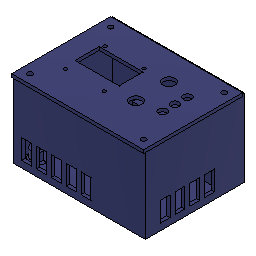
SensorUnit housing v20 (Autodesk Fusion 360 design; units mm, degrees)
Autodesk Fusion 360 part; units mm, degrees
sketch "Sketch1" plane through (0, 0, 0) normal (0, 1, 0) x (1, 0, 0)
  line L0 (26, -8.5) -> (-26, -8.5)
  line L1 (-26, -8.5) -> (-26, 8.5)
  line L2 (-26, 8.5) -> (26, 8.5)
  line L3 (26, 8.5) -> (26, -8.5)
  line L4 (26, -8.5) -> (-26, 8.5) construction
  line L5 (-26, -8.5) -> (26, 8.5) construction
  line L6 (15, -1) -> (-15, -1)
  line L7 (-15, -1) -> (-15, 1)
  line L8 (-15, 1) -> (15, 1)
  line L9 (15, 1) -> (15, -1)
  line L10 (15, -1) -> (-15, 1) construction
  line L11 (-15, -1) -> (15, 1) construction
  circle A0 centre (15, 0) radius 3.365
  circle A1 centre (-15, 0) radius 3.365
  dimension "d1" = 52
  dimension "d2" = 17
  dimension "d3" = 6.73
  dimension "d4" = 6.73
  constraint horizontal L0
  constraint perpendicular L0 L1
  constraint parallel L0 L2
  constraint parallel L1 L3
  constraint coincident L4 origin
  constraint coincident L5 origin
  constraint horizontal L6
  constraint perpendicular L6 L7
  constraint parallel L6 L8
  constraint parallel L7 L9
  constraint coincident L10 origin
  constraint coincident L11 origin
  constraint midpoint L9 A0.centre
  constraint midpoint L7 A1.centre
  measures "d1" distance of L1.end L2.end
  measures "d2" distance of L0.start L2.end
  measures "d3" diameter of A0
  measures "d4" diameter of A1
sketch "Sketch2" plane through (0, 0, 0) normal (0, 1, 0) x (1, 0, 0)
  line L0 (40, -30) -> (-40, -30)
  line L1 (-40, -30) -> (-40, 30)
  line L2 (-40, 30) -> (40, 30)
  line L3 (40, 30) -> (40, -30)
  line L4 (40, -30) -> (-40, 30) construction
  line L5 (-40, -30) -> (40, 30) construction
  line L6 (26, -14) -> (-26, -14) construction
  line L7 (-26, -14) -> (-26, 14) construction
  line L8 (-26, 14) -> (26, 14) construction
  line L9 (26, 14) -> (26, -14) construction
  line L10 (26, -14) -> (-26, 14) construction
  line L11 (-26, -14) -> (26, 14) construction
  line L12 (1.4523, -7.9433) -> (-23.5477, -7.9433) construction
  line L13 (-23.5477, -7.9433) -> (-23.5477, 8.0567) construction
  line L14 (-23.5477, 8.0567) -> (1.4523, 8.0567) construction
  line L15 (1.4523, 8.0567) -> (1.4523, -7.9433) construction
  line L16 (1.4523, -7.9433) -> (-23.5477, 8.0567) construction
  line L17 (-23.5477, -7.9433) -> (1.4523, 8.0567) construction
  point P0 (-11.0477, 0.0567)
  dimension "d7" = 80
  dimension "d8" = 60
  dimension "d9" = 52
  dimension "d10" = 28
  dimension "d11" = 25
  dimension "d12" = 16
  constraint horizontal L0
  constraint perpendicular L0 L1
  constraint parallel L0 L2
  constraint parallel L1 L3
  constraint coincident L4 origin
  constraint coincident L5 origin
  constraint horizontal L6
  constraint perpendicular L6 L7
  constraint parallel L6 L8
  constraint parallel L7 L9
  constraint coincident L10 origin
  constraint coincident L11 origin
  constraint horizontal L12
  constraint perpendicular L12 L13
  constraint parallel L12 L14
  constraint parallel L13 L15
  constraint coincident L16 P0
  constraint coincident L17 P0
  measures "d7" distance of L1.end L2.end
  measures "d8" distance of L0.start L2.end
  measures "d9" distance of L7.end L8.end
  measures "d10" distance of L6.end L7.end
  measures "d11" distance of L13.end L14.end
  measures "d12" distance of L12.end L13.end
extrude "Extrude2" add sketch "Sketch2" along normal blind 2.5 makes body 1
sketch "Sketch3" plane through (0, 2.5, 0) normal (0, 1, 0) x (-1, 0, 0)
  line L0 (-40, -30) -> (40, -30)
  line L1 (40, -30) -> (40, 30)
  line L2 (40, 30) -> (-40, 30)
  line L3 (-40, 30) -> (-40, -30)
  line L4 (40, -30) -> (-40, 30) construction
  line L5 (-40, -30) -> (40, 30) construction
  line L6 (-16.7, 25) -> (35, 25)
  line L7 (35, 25) -> (35, -3)
  line L8 (35, -3) -> (-16.7, -3)
  line L9 (-16.7, -3) -> (-16.7, 25)
  line L10 (-16.7, 25) -> (35, -3) construction
  line L11 (35, 25) -> (-16.7, -3) construction
  circle A0 centre (32.7, -0.7) radius 2.3971
  line L12 (9.15, -3) -> (9.15, 25) construction
  line L13 (35, 11) -> (-16.7, 11) construction
  circle A1 centre (32.7, 22.7) radius 2.3971
  circle A2 centre (-14.4, -0.7) radius 2.3971
  circle A3 centre (-14.4, 22.7) radius 2.3971
  circle A4 centre (32.7, -0.7) radius 3.8971
  circle A5 centre (32.7, 22.7) radius 3.8971
  circle A6 centre (-14.4, -0.7) radius 3.8971
  circle A7 centre (-14.4, 22.7) radius 3.8971
  point P0 (9.15, 11)
  dimension "d18" = 51.7
  dimension "d22" = 28
  dimension "d23" = 2.3
  dimension "d24" = 2.3
  dimension "d25" = 5
  dimension "d26" = 5
  dimension "d27" = 1.5
  constraint coincident L0.end L1.start
  constraint coincident L2.end L3.start
  constraint coincident L0.start L3.end
  constraint coincident L1.end L2.start
  constraint horizontal L6
  constraint perpendicular L6 L7
  constraint parallel L6 L8
  constraint parallel L7 L9
  constraint coincident L10 P0
  constraint coincident L11 P0
  constraint midpoint L8 L12.start
  constraint midpoint L6 L12.end
  constraint midpoint L7 L13.start
  constraint midpoint L9 L13.end
  constraint symmetric A0 L13 A1
  constraint symmetric A0 L12 A2
  constraint symmetric L12 A1 A3
  constraint concentric A0 A4
  constraint symmetric L13 A4 A5
  constraint symmetric L12 A4 A6
  constraint symmetric L12 A5 A7
  measures "d18" distance of L7.end L8.end
  measures "d22" distance of L6.start L8.end
  measures "d23" distance of L8 A0.centre
  measures "d24" distance of L7 A0.centre
  measures "d25" distance of L1 L7
  measures "d26" distance of L2 L6
  measures "d27" distance of A0 A4
extrude "Extrude4" cut sketch "Sketch3" against normal up to surface (2 mm away) from surface at -0.5 contours L6 L9 A3 A7 | L6 L9 A3 | L6 A3 | L6 L9 A3 | L9 A3 | L6 L9 A3 A7 | L6 L7 A1 A5 | L6 L7 A1 A5 | L8 L9 A2 A6 | L8 L9 A2 A6 | L6 A1 | L6 L7 A1 | L8 L9 A2 | L9 A2 | L6 L7 A1 | L7 A1 | L7 L8 A0 A4 | L7 L8 A0 A4 | L8 L9 A2 | L8 A2 | L7 A0 | L7 L8 A0 | L8 A0 | L7 L8 A0 bodies 1
extrude "Extrude5" cut sketch "Sketch3" against normal up to surface (0.5 mm away) contours L6 A3 | L6 L9 A3 | L9 A3 | L6 A1 | L6 L7 A1 | L8 L9 A2 | L9 A2 | L7 A1 | L8 A2 | L7 A0 | L7 L8 A0 | L8 A0 picked at (-15.1667, 23.1388) picked at (32.4467, 23.7731) picked at (-13.7719, -0.5156) picked at (33.3362, -0.4496) bodies 1
extrude "Extrude6" add sketch "Sketch3" along normal blind 6.5 from surface at -0.5 contours L6 L9 A3 A7 | L6 L9 A3 | L6 L9 A3 A7 | L6 L7 A1 A5 | L6 L7 A1 A5 | L8 L9 A2 A6 | L8 L9 A2 A6 | L6 L7 A1 | L7 L8 A0 A4 | L7 L8 A0 A4 | L8 L9 A2 | L7 L8 A0 picked at (-16.2938, 24.5938) picked at (34.5938, 24.5938) picked at (-16.2938, -2.5938) picked at (34.5938, -2.5938) bodies 1
chamfer "Chamfer1" distance 1 angle 45 1 edges at (-29.0666, 2.5, 0.7092) on bodies 1
chamfer "Chamfer1" distance 1 angle 45 3 edges at (-29.0666, 2.5, 24.1092) (18.0334, 2.5, 24.1092) (18.0334, 2.5, 0.7092) on bodies 1
sketch "Sketch4" plane through (0, 2.5, 0) normal (0, 1, 0) x (-1, 0, 0)
  line L0 (-38, 28) -> (38, 28)
  line L1 (38, 28) -> (38, -28)
  line L2 (38, -28) -> (-38, -28)
  line L3 (-38, -28) -> (-38, 28)
  line L4 (-38, 28) -> (38, -28) construction
  line L5 (38, 28) -> (-38, -28) construction
  line L6 (-40, -30) -> (40, -30)
  line L7 (40, 30) -> (-40, 30)
  line L8 (-40, 30) -> (-40, -30)
  line L9 (40, -30) -> (40, 30)
  line L10 (30, 8.5) -> (38, 8.5) construction
  dimension "d42" = 2
  dimension "d43" = 2
  dimension "d44" = 2
  dimension "d45" = 2
  constraint horizontal L0
  constraint perpendicular L0 L1
  constraint parallel L0 L2
  constraint parallel L1 L3
  constraint coincident L4 origin
  constraint coincident L5 origin
  constraint coincident L1 L10.end
  constraint perpendicular L1 L10
  measures "d42" distance of L1 L9
  measures "d43" distance of L3 L8
  measures "d44" distance of L2 L6
  measures "d45" distance of L0 L7
sketch "Sketch18" plane through (0, 2.5, 0) normal (0, 1, 0) x (-1, 0, 0)
  circle A0 centre (-14.4, 22.7) radius 4.8971
  circle A1 centre (32.7, -0.7) radius 4.8971
  line L0 (-40, -30) -> (40, -30)
  line L1 (40, -30) -> (40, 30)
  line L2 (40, 30) -> (-40, 30)
  line L3 (-40, 30) -> (-40, -30)
  circle A2 centre (32.7, 22.7) radius 4.8971
  circle A3 centre (-14.4, -0.7) radius 4.8971
  line L4 (32.7, -0.7) -> (32.7, 0.8) construction
  line L5 (32.7, 0.8) -> (28.0383, 0.8)
  line L6 (32.7, 0.8) -> (28.0383, 0.8)
  line L7 (32.7, 22.7) -> (32.7, 21.2) construction
  line L8 (32.7, 21.2) -> (28.0383, 21.2)
  line L9 (32.7, 21.2) -> (28.0383, 21.2)
  line L10 (32.7, 22.7) -> (27.8029, 22.7)
  line L11 (32.7, 22.7) -> (37.5971, 22.7)
  line L12 (32.7, -0.7) -> (27.8029, -0.7)
  line L13 (32.7, -0.7) -> (37.5971, -0.7)
  dimension "d140" = 1.5
  dimension "d141" = 1.5
  constraint coincident A1.centre L4.start
  constraint vertical L4
  constraint coincident A1 L5.end
  constraint perpendicular L4 L5
  constraint perpendicular L4 L6
  constraint coincident A2.centre L7.start
  constraint perpendicular L6 L7
  constraint coincident A2 L8.end
  constraint perpendicular L7 L8
  constraint perpendicular L7 L9
  constraint coincident A2 L10.end
  constraint perpendicular L7 L10
  constraint coincident A2 L11.end
  constraint perpendicular L7 L11
  constraint coincident A1 L12.end
  constraint perpendicular L4 L12
  constraint coincident A1 L13.end
  constraint perpendicular L4 L13
  measures "d140" distance of A1.centre L4.end
  measures "d141" distance of A2.centre L7.end
extrude "Extrude21" cut sketch "Sketch18" along normal up to surface (6 mm away) contours A1 L12 L13 | A2 L10 L11 picked at (32.7218, 2.5556) picked at (32.7218, 19.4444) bodies 1
extrude "Extrude7" add sketch "Sketch4" along normal blind 45 from surface at -0.5 bodies 1
sketch "Sketch5" plane through (0, 2.5, 0) normal (0, 1, 0) x (-1, 0, 0)
  line L0 (-38, -28) -> (13, -28)
  line L1 (13, -28) -> (13, -17)
  line L2 (13, -17) -> (-38, -17)
  line L3 (-38, -17) -> (-38, -28)
  line L4 (-38, -28) -> (14, -28)
  line L5 (14, -28) -> (14, -16)
  line L6 (14, -16) -> (-38, -16)
  line L7 (-38, -16) -> (-38, -28)
  line L8 (-40, 30) -> (-40, -30)
  line L9 (-40, -30) -> (40, -30)
  dimension "d49" = 51
  dimension "d50" = 11
  dimension "d51" = 1
  dimension "d52" = 1
  dimension "d215" = 2
  dimension "d216" = 2
  constraint horizontal L0
  constraint vertical L1
  constraint horizontal L2
  constraint vertical L3
  constraint horizontal L4
  constraint vertical L5
  constraint horizontal L6
  constraint vertical L7
  measures "d49" distance of L1.end L2.end
  measures "d50" distance of L0.end L1.end
  measures "d51" distance of L2 L6
  measures "d52" distance of L1 L5
  measures "d215" distance of L3 L8
  measures "d216" distance of L4 L9
extrude "Extrude8" add sketch "Sketch5" along normal blind 20 from surface at -0.5 contours L1 L2 L4 L5 L6 L7 bodies 1
sketch "Sketch6" plane through (0, 0, -28) normal (0, 0, 1) x (1, 0, 0)
  line L0 (-13, 2.5) -> (38, 2.5)
  line L1 (38, 2.5) -> (38, 47)
  line L2 (38, 47) -> (-38, 47)
  line L3 (-38, 47) -> (-38, 2.5)
  line L4 (38, 2.5) -> (-13, 2.5)
  line L5 (-13, 2.5) -> (-13, 22)
  line L6 (-13, 22) -> (38, 22)
  line L7 (38, 22) -> (38, 2.5)
  line L8 (36.5, 4) -> (-11.5, 4)
  line L9 (-11.5, 4) -> (-11.5, 20)
  line L10 (-11.5, 20) -> (36.5, 20)
  line L11 (36.5, 20) -> (36.5, 4)
  line L12 (-13, 22) -> (-13, 2.5)
  line L13 (-38, 2.5) -> (-14, 2.5)
  line L14 (-14, 2.5) -> (-14, 22)
  line L15 (-14, 22) -> (-13, 22)
  dimension "d56" = 1.5
  dimension "d57" = 1.5
  dimension "d58" = 1.5
  dimension "d59" = 16
  constraint horizontal L4
  constraint vertical L5
  constraint horizontal L6
  constraint vertical L7
  constraint coincident L0.end L1.start
  constraint horizontal L8
  constraint vertical L9
  constraint horizontal L10
  constraint vertical L11
  measures "d56" distance of L4 L8
  measures "d57" distance of L7 L11
  measures "d58" distance of L5 L9
  measures "d59" distance of L8 L10
extrude "Extrude9" cut sketch "Sketch6" against normal up to surface (2 mm away) contours L8 L9 L10 L11 bodies 1
sketch "Sketch7" plane through (0, 22, 0) normal (0, 1, 0) x (-1, 0, 0)
  line L0 (14, -28) -> (14, -16)
  line L1 (14, -16) -> (-38, -16)
  line L2 (-38, -17) -> (13, -17)
  line L3 (13, -17) -> (13, -28)
  line L4 (13, -25.5) -> (14, -25.5)
  line L5 (14, -25.5) -> (14, -17)
  line L6 (14, -17) -> (13, -17)
  line L7 (13, -17) -> (13, -25.5)
  line L8 (14, -16) -> (-38, -16)
  line L9 (-38, -16) -> (-38, -28)
  line L10 (-38, -28) -> (14, -28)
  line L11 (14, -28) -> (14, -16)
  line L12 (13, -28) -> (14, -28)
  line L13 (-38, -16) -> (-38, -17)
  line L14 (-40, -30) -> (40, -30)
  line L15 (-40, 30) -> (-40, -30)
  dimension "d63" = 8.5
  dimension "d217" = 2
  dimension "d218" = 2
  constraint horizontal L4
  constraint vertical L5
  constraint horizontal L6
  constraint vertical L7
  constraint coincident L0 L5.end
  constraint coincident L3 L4.start
  constraint horizontal L8
  constraint vertical L9
  constraint horizontal L10
  constraint vertical L11
  constraint coincident L0.end L1.start
  measures "d63" distance of L4.start L2.end
  measures "d217" distance of L10 L14
  measures "d218" distance of L9 L15
extrude "Extrude11" add sketch "Sketch7" along normal blind 1 from surface at -0.5 bodies 1
extrude "Extrude10" cut sketch "Sketch7" against normal blind 4 from surface at -0.5 contours L0 L3 L4 L5 L6 L7 L11 bodies 1
sketch "Sketch9" plane through (-38, 0, 0) normal (1, 0, 0) x (0, 0, -1)
  line L0 (-28, 2.5) -> (28, 2.5)
  line L1 (28, 2.5) -> (28, 47)
  line L2 (28, 47) -> (-28, 47)
  line L3 (-28, 47) -> (-28, 2.5)
  line L4 (-4.5, 3.5) -> (-17.5, 3.5)
  line L5 (-17.5, 3.5) -> (-17.5, 13.5)
  line L6 (-17.5, 13.5) -> (-4.5, 13.5)
  line L7 (-4.5, 13.5) -> (-4.5, 3.5)
  line L8 (-4.5, 3.5) -> (-17.5, 13.5) construction
  line L9 (-17.5, 3.5) -> (-4.5, 13.5) construction
  line L10 (-30, 0) -> (-30, 47)
  line L11 (-28, 2.5) -> (28, 2.5)
  point P0 (-11, 8.5)
  dimension "d71" = 19
  dimension "d72" = 6
  dimension "d73" = 10
  dimension "d74" = 13
  constraint horizontal L4
  constraint perpendicular L4 L5
  constraint parallel L4 L6
  constraint parallel L5 L7
  constraint coincident L8 P0
  constraint coincident L9 P0
  measures "d71" distance of P0 L10
  measures "d72" distance of P0 L11
  measures "d73" distance of L4 L6
  measures "d74" distance of L5.end L6.end
extrude "Extrude12" cut sketch "Sketch9" against normal up to surface (2 mm away) contours L4 L5 L6 L7 bodies 1
sketch "Sketch10" plane through (0, 47, 0) normal (0, 1, 0) x (-1, 0, 0)
  line L0 (38, -28) -> (-38, -28)
  line L1 (-38, -28) -> (-38, 28)
  line L2 (-38, 28) -> (38, 28)
  line L3 (38, 28) -> (38, -28)
  line L4 (40, -30) -> (40, 30)
  line L5 (40, 30) -> (-40, 30)
  line L6 (-40, 30) -> (-40, -30)
  line L7 (-40, -30) -> (40, -30)
  line L8 (-38, -28) -> (-30.9289, -20.9289)
  line L9 (-38, -28) -> (-23, -28) construction
  line L10 (-30.9289, -20.9289) -> (-38, -13.8579)
  line L11 (-30.9289, -20.9289) -> (-35.9289, -20.9289) construction
  line L12 (-30.9289, -20.9289) -> (-23.8579, -28)
  line L13 (0, -28) -> (0, 28) construction
  line L14 (-38, 28) -> (38, -28) construction
  line L15 (38, 0) -> (-38, 0) construction
  line L16 (-30.9289, 20.9289) -> (-38, 13.8579)
  line L17 (-30.9289, 20.9289) -> (-23.8579, 28)
  line L18 (30.9289, -20.9289) -> (38, -13.8579)
  line L19 (30.9289, -20.9289) -> (23.8579, -28)
  line L20 (30.9289, 20.9289) -> (38, 13.8579)
  line L21 (30.9289, 20.9289) -> (23.8579, 28)
  circle A0 centre (-34.4645, -24.4645) radius 1.5
  circle A1 centre (-34.4645, 24.4645) radius 1.5
  circle A2 centre (34.4645, -24.4645) radius 1.5
  circle A3 centre (34.4645, 24.4645) radius 1.5
  dimension "d78" = 45
  dimension "d79" = 10
  dimension "d80" = 45
  dimension "d81" = 180
  dimension "d85" = 3
  dimension "d86" = 5
  constraint horizontal L9
  constraint coincident L0.end L1.start
  constraint horizontal L11
  constraint coincident L1 L10.end
  constraint coincident L0 L12.end
  constraint midpoint L0 L13.start
  constraint midpoint L2 L13.end
  constraint coincident L1.end L2.start
  constraint coincident L0.start L3.end
  constraint midpoint L3 L15.start
  constraint midpoint L1 L15.end
  constraint symmetric L8.end L15 L16.start
  constraint symmetric L10.end L15 L16.end
  constraint symmetric L12.end L15 L17.end
  constraint symmetric L8.end L13 L18.start
  constraint symmetric L10.end L13 L18.end
  constraint symmetric L12.end L13 L19.end
  constraint symmetric L13 L16.start L20.start
  constraint symmetric L13 L16.end L20.end
  constraint symmetric L13 L17.end L21.end
  constraint coincident L8 A0.centre
  constraint symmetric L15 A0 A1
  constraint symmetric L13 A0 A2
  constraint symmetric L13 A1 A3
  measures "d78" angle of L8 L9
  measures "d79" distance of L0.end L8.end
  measures "d80" angle of L10 L11
  measures "d81" angle of L10 L12
  measures "d85" diameter of A0
  measures "d86" distance of L0.end A0.centre
extrude "Extrude13" add sketch "Sketch10" against normal blind 3 contours L0 L3 L18 L19 | L0 L8 L12 A0 | L2 L3 L20 L21 | L1 L8 L10 A0 | L8 A0 | L8 A0 | L1 L2 L16 L17 | A1 | A2 | A3 bodies 1
extrude "Extrude14" cut sketch "Sketch10" against normal up to surface (3 mm away) contours L8 A0 | L8 A0 | A1 | A2 | A3 bodies 1
sketch "Sketch11" plane through (0, 47, 0) normal (0, 1, 0) x (-1, 0, 0)
  line L0 (38.6239, -27.551) -> (-41.3761, -27.551)
  line L1 (-41.3761, -27.551) -> (-41.3761, 32.449)
  line L2 (-41.3761, 32.449) -> (38.6239, 32.449)
  line L3 (38.6239, 32.449) -> (38.6239, -27.551)
  line L4 (-1.3761, -27.551) -> (-1.3761, 32.449) construction
  line L5 (-41.3761, 2.449) -> (38.6239, 2.449) construction
  line L6 (36.6239, -25.551) -> (40.6239, -25.551) construction
  line L7 (40.6239, -25.551) -> (40.6239, -29.551) construction
  line L8 (40.6239, -29.551) -> (36.6239, -29.551) construction
  line L9 (36.6239, -29.551) -> (36.6239, -25.551) construction
  line L10 (36.6239, -25.551) -> (40.6239, -29.551) construction
  line L11 (40.6239, -25.551) -> (36.6239, -29.551) construction
  line L12 (36.6239, -25.551) -> (33.0884, -22.0155) construction
  line L13 (36.6239, -25.551) -> (28, -25.551) construction
  circle A0 centre (33.0884, -22.0155) radius 1.5
  circle A1 centre (-35.8405, -22.0155) radius 1.5
  circle A2 centre (-35.8405, 26.9134) radius 1.5
  circle A3 centre (33.0884, 26.9134) radius 1.5
  point P0 (38.6239, -27.551)
  dimension "d91" = 80
  dimension "d92" = 60
  dimension "d93" = 2
  dimension "d94" = 2
  dimension "d95" = 45
  dimension "d96" = 5
  dimension "d97" = 3
  constraint horizontal L0
  constraint vertical L1
  constraint horizontal L2
  constraint vertical L3
  constraint midpoint L0 L4.start
  constraint midpoint L2 L4.end
  constraint midpoint L1 L5.start
  constraint midpoint L3 L5.end
  constraint horizontal L6
  constraint perpendicular L6 L7
  constraint parallel L6 L8
  constraint parallel L7 L9
  constraint coincident L10 P0
  constraint coincident L11 P0
  constraint coincident P0 L0.start
  constraint horizontal L13
  constraint coincident L12.end A0.centre
  constraint symmetric L4 A0 A1
  constraint symmetric L5 A0 A3
  constraint symmetric L5 A1 A2
  measures "d91" distance of P0 L0.end
  measures "d92" distance of P0 L2.end
  measures "d93" distance of L3 L9
  measures "d94" distance of L0 L6
  measures "d95" angle of L12 L13
  measures "d96" distance of L6.start L12.end
  measures "d97" diameter of A0
extrude "Extrude15" add sketch "Sketch11" along normal blind 2 separate body makes body 2
sketch "Sketch12" plane through (0, 49, 0) normal (0, 1, 0) x (-1, 0, 0)
  circle A0 centre (33.0884, 26.9134) radius 1.5
  circle A1 centre (-35.8405, 26.9134) radius 1.5
  circle A2 centre (33.0884, -22.0155) radius 1.5
  circle A3 centre (-35.8405, -22.0155) radius 1.5
  line L0 (38.6239, 32.449) -> (-41.3761, 32.449)
  line L1 (-41.3761, 32.449) -> (-41.3761, -27.551)
  line L2 (-41.3761, -27.551) -> (38.6239, -27.551)
  line L3 (38.6239, -27.551) -> (38.6239, 32.449)
  line L4 (-0.35, 6.3) -> (26.35, 6.3)
  line L5 (26.35, 6.3) -> (26.35, -8.3)
  line L6 (26.35, -8.3) -> (-0.35, -8.3)
  line L7 (-0.35, -8.3) -> (-0.35, 6.3)
  line L8 (-0.35, 6.3) -> (26.35, -8.3) construction
  line L9 (26.35, 6.3) -> (-0.35, -8.3) construction
  line L10 (-0.7, 15.6) -> (26.7, 15.6) construction
  line L11 (26.7, 15.6) -> (26.7, -12.3) construction
  line L12 (26.7, -12.3) -> (-0.7, -12.3) construction
  line L13 (-0.7, -12.3) -> (-0.7, 15.6) construction
  line L14 (-0.7, 15.6) -> (26.7, -12.3) construction
  line L15 (26.7, 15.6) -> (-0.7, -12.3) construction
  line L16 (13, -12.3) -> (13, 15.6) construction
  circle A4 centre (1.3, -10.3) radius 1
  circle A5 centre (24.7, -10.3) radius 1
  line L17 (-0.7, 1.65) -> (26.7, 1.65) construction
  circle A6 centre (24.7, 13.6) radius 1
  circle A7 centre (1.3, 13.6) radius 1
  point P0 (13, -1)
  point P1 (13, 1.65)
  dimension "d101" = 14.6
  dimension "d102" = 26.7
  dimension "d103" = 27.4
  dimension "d104" = 27.9
  dimension "d105" = 4
  dimension "d106" = 2
  dimension "d107" = 2
  dimension "d108" = 2
  constraint horizontal L4
  constraint perpendicular L4 L5
  constraint parallel L4 L6
  constraint parallel L5 L7
  constraint coincident L8 P0
  constraint coincident L9 P0
  constraint horizontal L10
  constraint perpendicular L10 L11
  constraint parallel L10 L12
  constraint parallel L11 L13
  constraint coincident L14 P1
  constraint coincident L15 P1
  constraint midpoint L12 L16.start
  constraint midpoint L10 L16.end
  constraint coincident P0 L16
  constraint symmetric L16 A4 A5
  constraint midpoint L13 L17.start
  constraint midpoint L11 L17.end
  constraint symmetric A4 L17 A7
  constraint symmetric A5 L17 A6
  measures "d101" distance of L4.start L6.end
  measures "d102" distance of L4.start L4.end
  measures "d103" distance of L11.end L12.end
  measures "d104" distance of L10.start L12.end
  measures "d105" distance of L6 L12
  measures "d106" diameter of A4
  measures "d107" distance of L12 A4.centre
  measures "d108" distance of L13 A4.centre
extrude "Extrude16" cut sketch "Sketch12" against normal up to surface (2 mm away) contours L4 L5 L6 L7 | A4 | A5 | A6 | A7 bodies 2
sketch "Sketch13" plane through (0, 2.5, 0) normal (0, 1, 0) x (-1, 0, 0)
  circle A0 centre (-13.35, -11) radius 3.65
  circle A1 centre (-13.35, 9) radius 3.65
  line L0 (-0.35, -8.3) -> (-0.35, 6.3)
  line L1 (-0.35, -1) -> (-38.1982, -1) construction
  dimension "d112" = 7.3
  dimension "d113" = 7.3
  dimension "d114" = 20
  dimension "d115" = 13
  dimension "d116" = 10
  constraint midpoint L0 L1.start
  constraint perpendicular L0 L1
  measures "d112" diameter of A1
  measures "d113" diameter of A0
  measures "d114" distance of A0.centre A1.centre
  measures "d115" distance of A0.centre L0
  measures "d116" distance of A0.centre L1
extrude "Extrude17" cut sketch "Sketch13" along normal up to surface (46.5 mm away) bodies 2
sketch "Sketch14" plane through (0, 0, -17) normal (0, 0, -1) x (-1, 0, 0)
  line L0 (13, 21.5) -> (-38, 21.5)
  line L1 (-38, 2.5) -> (13, 2.5)
  line L2 (13, 2.5) -> (13, 17)
  circle A0 centre (-33.5, 11.5) radius 1
  line L3 (11.5, 4) -> (-36.5, 4)
  line L4 (-36.5, 4) -> (-36.5, 20)
  line L5 (-38, 21.5) -> (-38, 2.5)
  line L6 (13, 17) -> (14, 17)
  line L7 (14, 17) -> (14, 21)
  line L8 (14, 21) -> (13, 21)
  line L9 (13, 21) -> (13, 21.5)
  dimension "d120" = 2
  dimension "d121" = 7.5
  dimension "d122" = 3
  measures "d120" diameter of A0
  measures "d121" distance of A0.centre L3
  measures "d122" distance of A0.centre L4
extrude "Extrude18" cut sketch "Sketch14" against normal up to surface (1 mm away) contours A0 bodies 1
sketch "Sketch16" plane through (0, 49, 0) normal (0, 1, 0) x (-1, 0, 0)
  circle A0 centre (-13.35, 9) radius 3.65
  circle A1 centre (-13.35, -11) radius 3.65
  circle A2 centre (24.7, -10.3) radius 1
  circle A3 centre (1.3, -10.3) radius 1
  circle A4 centre (24.7, 13.6) radius 1
  line L0 (-0.35, -8.3) -> (-0.35, 6.3)
  line L1 (-0.35, 6.3) -> (26.35, 6.3)
  line L2 (26.35, 6.3) -> (26.35, -8.3)
  line L3 (26.35, -8.3) -> (-0.35, -8.3)
  circle A5 centre (1.3, 13.6) radius 1
  circle A6 centre (33.0884, 26.9134) radius 1.5
  circle A7 centre (-35.8405, 26.9134) radius 1.5
  circle A8 centre (33.0884, -22.0155) radius 1.5
  circle A9 centre (-35.8405, -22.0155) radius 1.5
  line L4 (38.6239, 32.449) -> (-41.3761, 32.449)
  line L5 (-41.3761, 32.449) -> (-41.3761, -27.551)
  line L6 (-41.3761, -27.551) -> (38.6239, -27.551)
  line L7 (38.6239, -27.551) -> (38.6239, 32.449)
  line L8 (-27, -13.193) -> (-27, 11.193) construction
  circle A10 centre (-27, -1) radius 2.5
  circle A11 centre (-27, -8.5) radius 2.5
  circle A12 centre (-27, 6.5) radius 2.5
  dimension "d133" = 5
  dimension "d134" = 5
  dimension "d135" = 5
  dimension "d136" = 7.5
  dimension "d137" = 7.5
  constraint vertical L8
  constraint midpoint L8 A10.centre
  constraint coincident L8 A11.centre
  constraint coincident L8 A12.centre
  measures "d133" diameter of A10
  measures "d134" diameter of A11
  measures "d135" diameter of A12
  measures "d136" distance of A10.centre A12.centre
  measures "d137" distance of A10.centre A11.centre
extrude "Extrude20" cut sketch "Sketch16" against normal up to surface (2 mm away) contours A10 | A11 | A12 bodies 2
sketch "Sketch19" plane through (40, 0, 0) normal (1, 0, 0) x (0, 0, -1)
  line L0 (-30, 47) -> (-30, 0)
  line L1 (-30, 0) -> (30, 0)
  line L2 (30, 0) -> (30, 47)
  line L3 (30, 47) -> (-30, 47)
  line L4 (30, 10) -> (-30, 10) construction
  line L5 (3, 16) -> (-3, 16)
  line L6 (-3, 16) -> (-3, 4)
  line L7 (-3, 4) -> (3, 4)
  line L8 (3, 4) -> (3, 16)
  line L9 (3, 16) -> (-3, 4) construction
  line L10 (-3, 16) -> (3, 4) construction
  line L11 (12, 16) -> (6, 16)
  line L12 (6, 16) -> (6, 4)
  line L13 (6, 4) -> (12, 4)
  line L14 (12, 4) -> (12, 16)
  line L15 (12, 16) -> (6, 4) construction
  line L16 (6, 16) -> (12, 4) construction
  line L17 (0, 0) -> (0, 16) construction
  line L18 (-6, 16) -> (-6, 4)
  line L19 (-12, 16) -> (-6, 16)
  line L20 (-12, 4) -> (-12, 16)
  line L21 (-6, 4) -> (-12, 4)
  line L22 (-15, 16) -> (-15, 4)
  line L23 (-21, 16) -> (-15, 16)
  line L24 (-21, 4) -> (-21, 16)
  line L25 (-15, 4) -> (-21, 4)
  point P0 (0, 10)
  point P1 (9, 10)
  point P2 (18, 10)
  point P3 (-27, 10)
  dimension "d146" = 10
  dimension "d147" = 6
  dimension "d148" = 12
  dimension "d149" = 6
  dimension "d150" = 12
  dimension "d151" = 3
  constraint coincident L2 L4.start
  constraint coincident L0 L4.end
  constraint perpendicular L0 L4
  constraint horizontal L5
  constraint perpendicular L5 L6
  constraint parallel L5 L7
  constraint parallel L6 L8
  constraint coincident L9 P0
  constraint coincident L10 P0
  constraint midpoint L4 P0
  constraint horizontal L11
  constraint perpendicular L11 L12
  constraint parallel L11 L13
  constraint parallel L12 L14
  constraint coincident L15 P1
  constraint coincident L16 P1
  constraint coincident L4 P1
  constraint coincident L4 P2
  constraint coincident L17.start origin
  constraint midpoint L5 L17.end
  constraint symmetric L11.start L17 L19.start
  constraint symmetric L11.end L17 L18.start
  constraint symmetric L12.end L17 L18.end
  constraint symmetric L13.end L17 L20.start
  constraint coincident L4 P3
  measures "d146" distance of L1 L4
  measures "d147" distance of L6.end L7.end
  measures "d148" distance of L5.end L6.end
  measures "d149" distance of L12.end L13.end
  measures "d150" distance of L11.end L12.end
  measures "d151" distance of L8 L12
extrude "Extrude22" cut sketch "Sketch19" against normal up to surface (2 mm away) contours L5 L6 L7 L8 | L11 L12 L13 L14 | L18 L19 L20 L21 | L22 L23 L24 L25 bodies 1
sketch "Sketch20" plane through (0, 0, 30) normal (0, 0, 1) x (1, 0, 0)
  line L0 (-40, 47) -> (-40, 0)
  line L1 (-40, 0) -> (40, 0)
  line L2 (40, 0) -> (40, 47)
  line L3 (40, 47) -> (-40, 47)
  line L4 (-40, 10) -> (40, 10) construction
  line L5 (-2, 4) -> (-8, 4)
  line L6 (-8, 4) -> (-8, 16)
  line L7 (-8, 16) -> (-2, 16)
  line L8 (-2, 16) -> (-2, 4)
  line L9 (-2, 4) -> (-8, 16) construction
  line L10 (-8, 4) -> (-2, 16) construction
  line L11 (7, 4) -> (1, 4)
  line L12 (1, 4) -> (1, 16)
  line L13 (1, 16) -> (7, 16)
  line L14 (7, 16) -> (7, 4)
  line L15 (7, 4) -> (1, 16) construction
  line L16 (1, 4) -> (7, 16) construction
  line L17 (-5, 16) -> (-5, 4) construction
  line L18 (-35, 16) -> (-35, 4)
  line L19 (-29, 16) -> (-35, 16)
  line L20 (-29, 4) -> (-29, 16)
  line L21 (-35, 4) -> (-29, 4)
  line L22 (-26, 16) -> (-26, 4)
  line L23 (-26, 4) -> (-20, 4)
  line L24 (-20, 4) -> (-20, 16)
  line L25 (-20, 16) -> (-26, 16)
  line L26 (-17, 16) -> (-17, 4)
  line L27 (-11, 16) -> (-17, 16)
  line L28 (-11, 4) -> (-11, 16)
  line L29 (-17, 4) -> (-11, 4)
  point P0 (-5, 10)
  point P1 (4, 10)
  point P2 (-5, 4)
  point P3 (-5, 16)
  point P4 (-8, 4)
  point P5 (-2, 4)
  point P6 (-2, 16)
  point P7 (-5, 10)
  dimension "d163" = 10
  dimension "d164" = 6
  dimension "d165" = 12
  dimension "d166" = 6
  dimension "d167" = 12
  dimension "d170" = 3
  dimension "d175" = 5
  dimension "d219" = 6
  dimension "d220" = 3
  dimension "d221" = 3
  dimension "d222" = 6
  constraint horizontal L4
  constraint coincident L0 L4.start
  constraint coincident L2 L4.end
  constraint horizontal L5
  constraint perpendicular L5 L6
  constraint parallel L5 L7
  constraint parallel L6 L8
  constraint coincident L9 P7
  constraint coincident L10 P7
  constraint coincident L4 P7
  constraint horizontal L11
  constraint perpendicular L11 L12
  constraint parallel L11 L13
  constraint parallel L12 L14
  constraint coincident L15 P1
  constraint coincident L16 P1
  constraint coincident L4 P1
  constraint vertical L17
  constraint midpoint L7 P3
  constraint coincident L5 P2
  constraint symmetric P5 L17 P4
  constraint symmetric P4 L17 P5
  constraint symmetric L6.end L17 P6
  constraint symmetric P7 L17 P0
  constraint symmetric L11.start L17 L26.end
  constraint symmetric L11.end L17 L28.start
  constraint symmetric L12.end L17 L27.start
  constraint symmetric L13.end L17 L26.start
  constraint symmetric P3 L17 L17.start
  constraint symmetric P2 L17 L17.end
  measures "d163" distance of L1 L4
  measures "d164" distance of L6.end P6
  measures "d165" distance of P4 L6.end
  measures "d166" distance of L12.end L13.end
  measures "d167" distance of L11.end L12.end
  measures "d170" distance of L8 L12
  measures "d175" distance of L0 L18
  measures "d219" distance of L18.start L19.start
  measures "d220" distance of L20 L22
  measures "d221" distance of L24 L26
  measures "d222" distance of L22.start L24.end
extrude "Extrude23" cut sketch "Sketch20" against normal up to surface (2 mm away) contours L5 L6 L7 L8 | L11 L12 L13 L14 | L18 L19 L20 L21 | L22 L23 L24 L25 | L26 L27 L28 L29 bodies 1
equation "d23 = 0.8 mm + 1.5 mm"
equation "d116 = 6.5 mm + 3.5 mm"
named bodies: "casing body", "casing lid"
